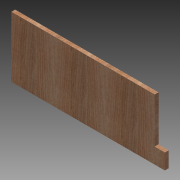
# Autodesk Inventor part: Shooter_Mount
Saved by Autodesk Inventor 2014 (Build 180170000, 170)
## iProperties
Created: 2016-01-28
Part Number: Shooter_Mount
Material: Generic
Document SubType Name: Modeling
Designer: choices
Density: 1 g/cm^3
Appearance: Birch - Natural Polished
Author: choices
Autodesk Inventor part; units mm, degrees
ref_plane "YZ Plane" through (0, 0, 0) normal (1, 0, 0) x (0, 1, 0)
ref_plane "XZ Plane" through (0, 0, 0) normal (0, 1, 0) x (-1, 0, 0)
ref_plane "XY Plane" through (0, 0, 0) normal (0, 0, 1) x (1, 0, 0)
sketch "Sketch1" plane through (0, 0, 0) normal (0, 0, 1) x (1, 0, 0)
  line L0 (-82.725, 0) -> (687.911, 0)
  line L1 (687.911, 0) -> (687.911, 78.232)
  line L2 (687.911, 78.232) -> (637.111, 78.232)
  line L3 (637.111, 78.232) -> (637.111, 304.8)
  line L4 (637.111, 304.8) -> (-82.725, 304.8)
  line L5 (-82.725, 304.8) -> (-82.725, 0)
  point P0 (0, 0)
  dimension "d0" = 770.636
  dimension "d1" = 78.232
  dimension "d2" = 50.8
  dimension "d3" = 226.568
  constraints: 12 end point, 4 perpendicular, 1 horizontal, 1 parallel
  measures "d0" distance of L0.start L0.end
  measures "d1" distance of L0.end L1.end
  measures "d2" distance of L1.end L2.end
  measures "d3" distance of L2.end L3.end
extrude "Extrusion1" add sketch "Sketch1" along normal blind 19.05
body "Solid1"
